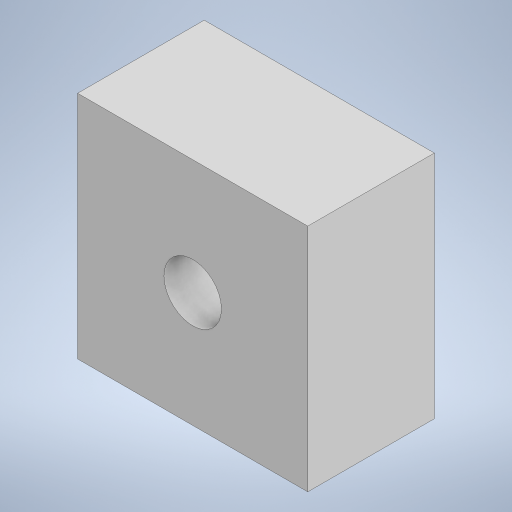
# Autodesk Inventor part: Touchscreen mount v04
Saved by Autodesk Inventor 2023 (Build 270158000, 158)
## iProperties
Created: 2024-06-29
Part Number: Touchscreen mount v04
Material: Generic
Document SubType Name: Modeling
Designer: Akramilab
Density: 1 g/cm^3
Appearance: Default
Author: Akramilab
Autodesk Inventor part; units mm, degrees
ref_plane "YZ Plane" through (0, 0, 0) normal (1, 0, 0) x (0, 1, 0)
ref_plane "XZ Plane" through (0, 0, 0) normal (0, 1, 0) x (-1, 0, 0)
ref_plane "XY Plane" through (0, 0, 0) normal (0, 0, 1) x (1, 0, 0)
sketch "Sketch1" plane through (0, 0, 0) normal (0, 0, 1) x (1, 0, 0)
  line L0 (0, 20) -> (20, 20)
  line L1 (20, 20) -> (20, 0)
  line L2 (20, 0) -> (0, 0)
  line L3 (0, 0) -> (0, 20)
  circle A0 centre (10, 10) radius 2.5
  dimension "d0" = 20
  dimension "d1" = 20
  dimension "d5" = 10
  dimension "d6" = 10
  dimension "d7" = 5
  constraints: 8 end point, 2 parallel, 1 centre point, 1 coincident, 1 horizontal, 1 perpendicular
  measures "d0" distance between parallel lines of L2 L0
  measures "d1" distance between parallel lines of L1 L3
  measures "d5" distance from line of point (10, 10) L3
  measures "d6" distance from line of L2 point (10, 10)
  measures "d7" diameter of A0
extrude "Extrusion2" add sketch "Sketch1" along normal blind 5
sketch "Sketch3" plane through (0, 0, 0) normal (0, 0, -1) x (-1, 0, 0)
  line L0 (-20, 20) -> (0, 20) projected
  line L1 (0, 20) -> (0, 0) projected
  line L2 (-20, 20) -> (0, 20)
  line L3 (0, 20) -> (0, 0)
  line L4 (0, 0) -> (-20, 0)
  line L5 (-20, 0) -> (-20, 20)
  circle A0 centre (-10, 10) radius 4.5
  dimension "d10" = 9
  constraints: 8 end point, 2 parallel, 1 centre point, 1 horizontal, 1 perpendicular
  measures "d10" diameter of A0
extrude "Extrusion3" add sketch "Sketch3" along normal blind 6
equation "\"d1\" = d0"
equation "\"d5\" = 0.5 * d0"
equation "\"d6\" = d5"
body "Solid2"
